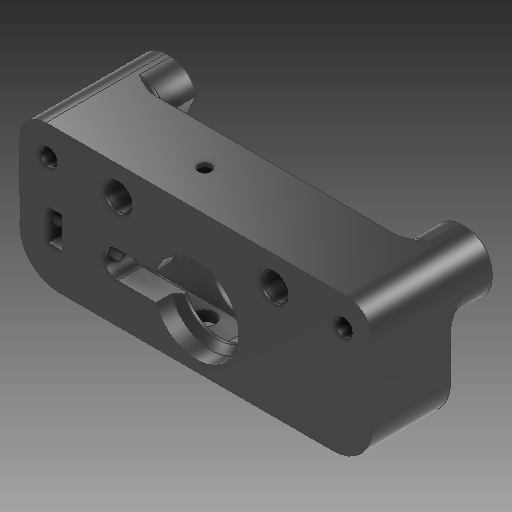
# Autodesk Inventor part: Extruder Clamp Block
Saved by Autodesk Inventor 2020.2 (Build 242310000, 310)
## iProperties
Created: 2020-03-19
Part Number: Extruder Clamp Block
Material: ABS Plastic
Document SubType Name: Modeling
Designer: rah75
Density: 1.06 g/cm^3
Appearance: Satin - Black
Author: rah75
Title: Upper Extruder Block
Autodesk Inventor part; units mm, degrees
ref_plane "YZ Plane" through (0, 0, 0) normal (1, 0, 0) x (0, 1, 0)
ref_plane "XZ Plane" through (0, 0, 0) normal (0, 1, 0) x (-1, 0, 0)
ref_plane "XY Plane" through (0, 0, 0) normal (0, 0, 1) x (1, 0, 0)
sketch "Sketch1" plane through (0, 0, 0) normal (0, 0, 1) x (1, 0, 0)
  line L0 (-28.9, 13) -> (28.9, 13)
  line L1 (33.9, 8) -> (33.9, -14)
  line L2 (33.9, -14) -> (-33.9, -14)
  line L3 (-33.9, -14) -> (-33.9, 8)
  arc A0 (33.9, 8) -> (28.9, 13) centre (28.9, 8) ccw
  arc A1 (-28.9, 13) -> (-33.9, 8) centre (-28.9, 8) ccw
  point P0 (0, 0)
  point P1 (-33.9, 13)
  point P2 (33.9, 13)
  point P3 (0, -14)
  point P4 (28.4, 7.5)
  point P5 (-28.4, 7.5)
  dimension "d2" = 27
  dimension "d72" = 67.8
  dimension "d73" = 5
  dimension "d74" = 57.8
  dimension "d75" = 14
  dimension "d76" = 5.5
  dimension "d77" = 5.5
  dimension "d78" = 5.5
  dimension "d79" = 5.5
  constraints: 8 end point, 4 point on circle, 4 point on line, 4 tangent, 2 centre point, 2 parallel, 1 equal radius, 1 horizontal, 1 midpoint, 1 perpendicular, 1 vertical alignment
  measures "d2" distance of L2.end point (-33.9, 13)
  measures "d72" distance of point (-33.9, 13) point (33.9, 13)
  measures "d73" radius of A0
  measures "d74" distance of A1.centre A0.centre
  measures "d75" distance from line of L2 point (0, 0)
  measures "d76" distance from line of L3 point (-28.4, 7.5)
  measures "d77" distance from line of L1 point (28.4, 7.5)
  measures "d78" distance from line of L0 point (28.4, 7.5)
  measures "d79" distance from line of L0 point (-28.4, 7.5)
extrude "Extrusion1" add sketch "Sketch1" along normal blind 15
fillet "Fillet1" radius 7.5 2 edges at (-33.9, -14, 7.5) (33.9, -14, 7.5)
sketch "Sketch10" plane through (0, 0, 0) normal (0, 0, -1) x (-1, 0, 0)
  arc A0 (-28.9, 13) -> (-33.9, 8) centre (-28.9, 8) ccw projected
  arc A1 (33.9, 8) -> (28.9, 13) centre (28.9, 8) ccw projected
  line L0 (-28.9, 13) -> (28.9, 13) projected
  line L1 (-33.9, -6.5) -> (-33.9, 8) projected
  line L2 (33.9, 8) -> (33.9, -6.5) projected
  point P0 (0, 0)
  point P1 (28.4, 7.5)
  point P2 (-28.4, 7.5)
  point P3 (-33.9, -13)
  point P4 (33.9, -13)
  dimension "d80" = 5.5
  dimension "d81" = 5.5
  dimension "d82" = 5.5
  dimension "d83" = 5.5
  measures "d80" distance from line of point (-28.4, 7.5) L0
  measures "d81" distance from line of L1 point (-28.4, 7.5)
  measures "d82" distance from line of point (28.4, 7.5) L0
  measures "d83" distance from line of L2 point (28.4, 7.5)
hole "Hole4" at (-28.4, 7.5, 0) at (28.4, 7.5, 0) direction (0, 0, 1) diameter 3.4 end through all clearance for "Socket Head Cap Screw" size "M3" standard "Ansi Metric M Profile"
sketch "Sketch2" plane through (-23.7815, 13, 0) normal (0, 1, 0) x (1, 0, 0)
  line L0 (52.6815, -15) -> (-5.1185, -15) projected
  point P0 (23.7815, 0)
  point P1 (17.6815, -7.25)
  dimension "d16" = 7.75
  dimension "d29" = 6.1
  measures "d16" distance from line of L0 point (17.682, -7.25)
  measures "d29" horizontal distance of point (17.682, -7.25) point (23.782, 0)
hole "Hole1" at (-6.1, 13, 7.25) direction (0, -1, 0) diameter 4 end through all
sketch "Sketch3" plane through (0, 0, 15) normal (0, 0, 1) x (1, 0, 0)
  circle A0 centre (0, -3.8) radius 7
  line L0 (33.9, -6.5) -> (33.9, 8) projected
  line L1 (28.9, 13) -> (-28.9, 13) projected
  point P0 (0, 0)
  point P1 (33.9, -1.1185)
  point P2 (21.2815, 11.5)
  point P3 (-21.2815, 11.5)
  point P4 (33.9, -13)
  dimension "d17" = 14
  dimension "d19" = 16.8
  constraints: 1 centre point, 1 vertical alignment, 1 other
  measures "d17" diameter of A0
extrude "Extrusion2" cut sketch "Sketch3" against normal blind 3.5
sketch "Sketch4" plane through (0, -3.8, 11.5) normal (0, 0, 1) x (1, 0, 0)
  circle A0 centre (0, 0) radius 7 projected
  point P0 (0, 3.8)
  point P1 (-4.2202, 6.2)
  point P2 (4.2202, 6.2)
  constraints: 1 coincident, 1 other
hole "Hole2" at (0, -3.8, 11.5) direction (0, 0, -1) diameter 11.5 end through all
sketch "Sketch5" plane through (0, 0, 0) normal (0, 0, -1) x (-1, 0, 0)
  circle A0 centre (0, -3.8) radius 5.75 projected
  line L0 (0, -3.8) -> (15.15, -3.8) construction
  line L1 (0, -6.425) -> (15.15, -6.425)
  line L2 (15.15, -1.175) -> (0, -1.175)
  arc A1 (0, -1.175) -> (0, -6.425) centre (0, -3.8) ccw
  arc A2 (15.15, -6.425) -> (15.15, -1.175) centre (15.15, -3.8) ccw
  point P0 (0, 0)
  point P1 (7.575, -3.8)
  dimension "d30" = 5.25
  dimension "d31" = 15.15
  constraints: 8 end point, 4 point on circle, 4 tangent, 2 centre point, 1 coincident, 1 horizontal, 1 midpoint, 1 parallel
  measures "d30" diameter of A2
  measures "d31" distance of L0.end A0.centre
extrude "Extrusion3" cut sketch "Sketch5" against normal through all contours A0 L1 A1 L2 | A0 L2 A2 L1 picked at (1.9167, -3.8)
sketch "Sketch6" plane through (0, 0, 0) normal (1, 0, 0) x (0, 1, 0)
  line L0 (-6.425, 15) -> (-1.175, 15) projected
  line L1 (-6.425, 0) -> (-6.425, 15) projected
  line L2 (-1.175, 0) -> (-6.425, 0) projected
  line L3 (-1.175, 0) -> (-1.175, 15) projected
  line L4 (4.45, 10.25) -> (-12.05, 10.25)
  line L5 (-12.05, 10.25) -> (-12.05, 4.25)
  line L6 (-12.05, 4.25) -> (4.45, 4.25)
  line L7 (4.45, 4.25) -> (4.45, 10.25)
  line L8 (4.45, 10.25) -> (-12.05, 4.25) construction
  line L9 (-12.05, 10.25) -> (4.45, 4.25) construction
  point P0 (0, 0)
  point P1 (-3.8, 7.25)
  point P2 (-3.8, 7.25)
  point P3 (-3.8, 0)
  dimension "d34" = 7.75
  dimension "d35" = 16.5
  dimension "d36" = 6
  constraints: 12 end point, 4 midpoint, 2 parallel, 1 horizontal, 1 perpendicular, 1 vertical alignment
  measures "d34" distance from line of L0 point (-3.8, 7.25)
  measures "d35" distance of L5.end L6.end
  measures "d36" distance of L6.end L4.start
extrude "Extrusion4" cut sketch "Sketch6" against normal blind 25 contours L4 L3 L6 L1 | L1 L6 L5 L4 | L4 L7 L6 L3
fillet "Fillet2" radius 8.25 2 edges at (-25, 4.45, 7.25) (-25, -12.05, 7.25)
sketch "Sketch7" plane through (0, 0, 0) normal (0, 0, -1) x (-1, 0, 0)
  arc A0 (5.1158, -1.175) -> (0, 1.95) centre (0, -3.8) ccw projected
  arc A1 (16.75, -12.05) -> (16.75, 4.45) centre (16.75, -3.8) ccw projected
  line L0 (0, 4.45) -> (16.75, 4.45) projected
  line L1 (0, 4.45) -> (0, 1.95) projected
  arc A2 (5.1158, -1.175) -> (0, 1.95) centre (0, -3.8) ccw projected
  line L2 (15.15, -1.175) -> (5.1158, -1.175) projected
  arc A3 (15.15, -6.425) -> (15.15, -1.175) centre (15.15, -3.8) ccw projected
  line L3 (5.1158, -6.425) -> (15.15, -6.425) projected
  arc A4 (0, -9.55) -> (5.1158, -6.425) centre (0, -3.8) ccw projected
  line L4 (0, -9.55) -> (0, -12.05) projected
  circle A5 centre (0, -3.8) radius 8.25
  line L5 (0, -12.05) -> (16.75, -12.05) projected
  point P0 (0, 0)
  constraints: 1 centre point, 1 coincident, 1 tangent
extrude "Extrusion5" cut sketch "Sketch7" against normal up to surface (10.25 mm away) contours L2 A5 L3 A4 L4 L1 A0 | A0 L1 A5 L2 | L4 A4 L3 A5
sketch "Sketch8" plane through (-33.9, -6.5, 0) normal (-1, 0, 0) x (0, 0, 1)
  line L0 (4.25, 0.075) -> (4.25, 5.325) projected
  line L1 (10.25, 5.325) -> (10.25, 0.075) projected
  line L2 (0, 0.075) -> (0, 5.325) projected
  line L3 (15, 5.325) -> (15, 0.075) projected
  line L4 (0, 2.7) -> (4.25, 2.7)
  line L5 (10.25, 2.7) -> (15, 2.7)
  point P0 (0, 6.5)
  point P1 (2.125, 2.7)
  point P2 (12.625, 2.7)
  point P3 (2.125, 2.7)
  point P4 (12.625, 2.7)
  constraints: 6 midpoint, 4 end point, 2 coincident, 2 horizontal
hole "Hole3" at (-33.9, -3.8, 2.125) at (-33.9, -3.8, 12.625) direction (1, 0, 0) diameter 3.2 end up to surface counterbore diameter 6.5 counterbore depth 0.1 clearance for "Socket Head Cap Screw" size "M3" standard "Ansi Metric M Profile"
sketch "Sketch9" plane through (0, 0, 0) normal (0, 0, -1) x (-1, 0, 0)
  line L0 (-28.9, 13) -> (28.9, 13) projected
  line L1 (-33.9, -6.5) -> (-33.9, 8) projected
  line L2 (26.4, -14) -> (-26.4, -14) projected
  arc A0 (7.8212, -1.175) -> (7.8212, -6.425) centre (0, -3.8) ccw projected
  line L3 (7.8212, -1.175) -> (15.15, -1.175) projected
  arc A1 (15.15, -6.425) -> (15.15, -1.175) centre (15.15, -3.8) ccw projected
  line L4 (15.15, -6.425) -> (7.8212, -6.425) projected
  line L5 (25.775, -0.8) -> (28.525, -0.8)
  line L6 (28.525, -0.8) -> (28.525, -6.8)
  line L7 (28.525, -6.8) -> (25.775, -6.8)
  line L8 (25.775, -6.8) -> (25.775, -0.8)
  line L9 (25.775, -0.8) -> (28.525, -6.8) construction
  line L10 (28.525, -0.8) -> (25.775, -6.8) construction
  line L11 (33.9, 8) -> (33.9, -1.341) projected
  arc A2 (33.9, 8) -> (28.9, 13) centre (28.9, 8) ccw projected
  arc A3 (-28.9, 13) -> (-33.9, 8) centre (-28.9, 8) ccw projected
  line L12 (33.8, -1.341) -> (33.9, -1.341) projected
  arc A4 (-33.9, -6.5) -> (-26.4, -14) centre (-26.4, -6.5) ccw projected
  arc A5 (26.4, -14) -> (33.9, -6.5) centre (26.4, -6.5) ccw projected
  line L13 (33.9, -6.259) -> (33.8, -6.259) projected
  line L14 (33.8, -6.259) -> (33.8, -1.341) projected
  line L15 (33.9, -6.259) -> (33.9, -6.5) projected
  point P0 (0, 0)
  point P1 (27.15, -3.8)
  point P2 (27.15, -3.8)
  point P3 (39.8, -3.8)
  point P4 (27.15, -3.8)
  dimension "d49" = 2.75
  dimension "d50" = 6
  dimension "d51" = 8
  constraints: 12 end point, 4 midpoint, 2 horizontal alignment, 2 parallel, 1 horizontal, 1 perpendicular
  measures "d49" distance of L5.start L5.end
  measures "d50" distance of L7.end L5.start
  measures "d51" distance edge to line of A1 L8
extrude "Extrusion6" cut sketch "Sketch9" against normal blind 21.1125 contours L5 L6 L7 L8
sketch "Sketch11" plane through (0, 0, 0) normal (0, 0, -1) x (-1, 0, 0)
  circle A0 centre (28.4, 7.5) radius 1.7 projected
  circle A1 centre (-28.4, 7.5) radius 1.7 projected
  line L0 (28.525, -0.8) -> (28.525, -6.8) projected
  line L1 (28.525, -6.8) -> (25.775, -6.8) projected
  line L2 (25.775, -6.8) -> (25.775, -0.8) projected
  line L3 (25.775, -0.8) -> (28.525, -0.8) projected
  line L4 (-28.9, 13) -> (28.9, 13) projected
  line L5 (-33.9, -6.5) -> (-33.9, 8) projected
  line L6 (26.4, -14) -> (-26.4, -14) projected
  arc A2 (7.8212, -1.175) -> (7.8212, -6.425) centre (0, -3.8) ccw projected
  line L7 (7.8212, -1.175) -> (15.15, -1.175) projected
  arc A3 (15.15, -6.425) -> (15.15, -1.175) centre (15.15, -3.8) ccw projected
  line L8 (15.15, -6.425) -> (7.8212, -6.425) projected
  circle A4 centre (-28.4, 7.5) radius 5.5
  circle A5 centre (28.4, 7.5) radius 1.7 projected
  circle A6 centre (28.4, 7.5) radius 5
  line L9 (33.9, 8) -> (33.9, -1.341) projected
  arc A7 (33.9, 8) -> (28.9, 13) centre (28.9, 8) ccw projected
  arc A8 (-28.9, 13) -> (-33.9, 8) centre (-28.9, 8) ccw projected
  line L10 (33.8, -1.341) -> (33.9, -1.341) projected
  arc A9 (-33.9, -6.5) -> (-26.4, -14) centre (-26.4, -6.5) ccw projected
  arc A10 (26.4, -14) -> (33.9, -6.5) centre (26.4, -6.5) ccw projected
  line L11 (33.9, -6.259) -> (33.8, -6.259) projected
  line L12 (33.8, -6.259) -> (33.8, -1.341) projected
  line L13 (22.9, 2) -> (33.9, 2)
  line L14 (33.9, 2) -> (33.9, 13)
  line L15 (33.9, 13) -> (22.9, 13)
  line L16 (22.9, 13) -> (22.9, 2)
  line L17 (22.9, 2) -> (33.9, 13) construction
  line L18 (33.9, 2) -> (22.9, 13) construction
  line L19 (33.9, 8) -> (33.9, -1.341) projected
  line L20 (-22.9, 2) -> (-33.9, 2)
  line L21 (-33.9, 2) -> (-33.9, 13)
  line L22 (-33.9, 13) -> (-22.9, 13)
  line L23 (-22.9, 13) -> (-22.9, 2)
  circle A11 centre (-28.4, 7.5) radius 1.7 projected
  line L24 (-22.9, 2) -> (-33.9, 13) construction
  line L25 (-33.9, 2) -> (-22.9, 13) construction
  line L26 (-33.9, -6.5) -> (-33.9, 8) projected
  line L27 (33.9, -6.259) -> (33.9, -6.5) projected
  point P0 (0, 0)
  point P1 (33.9, 8)
  point P2 (-22.9, 7.5)
  point P3 (-28.4, 13)
  point P4 (-28.4, 2)
  point P5 (-33.9, 7.5)
  point P6 (-33.9, 8)
  dimension "d61" = 11
  dimension "d62" = 10
  constraints: 24 end point, 4 collinear, 4 midpoint, 4 parallel, 2 centre point, 2 coincident, 2 horizontal, 2 perpendicular
  measures "d61" diameter of A4
  measures "d62" diameter of A6
extrude "Extrusion7" add sketch "Sketch11" along normal blind 8 contours L23 A4 L4 | L4 A7 L9 L13 L16 | A4 L5 A8 L4 | A4 | L23 L20 A4 | L15 L14 A7 | A8 L21 L22 | A4 L20 L5 | A6
fillet "Fillet4" radius 5 8 edges at (-33.9, 13, -4) (-22.9, 13, -4) (-33.9, 2, -4) (-22.9, 2, -4) (33.9, 13, -4) (33.9, 2, -4) (22.9, 2, -4) (22.9, 13, -4)
fillet "Fillet3" radius 2 10 edges at (22.9, 7.5, 0) (24.3645, 3.4645, 0) (28.4, 2, 0) (32.4355, 3.4645, 0) (24.3645, 11.5355, 0) (-24.3645, 11.5355, 0) (-24.3645, 3.4645, 0) (-28.4, 2, 0) (-32.4355, 3.4645, 0) (-22.9, 7.5, 0)
sketch "Sketch12" plane through (0, 0, 0) normal (0, 0, -1) x (-1, 0, 0)
  arc A0 (7.8212, -1.175) -> (7.8212, -6.425) centre (0, -3.8) ccw projected
  circle A1 centre (0, -3.8) radius 26.25
  dimension "d66" = 52.5
  constraints: 2 coincident, 1 centre point
  measures "d66" diameter of A1
extrude "Extrusion8" cut sketch "Sketch12" along normal blind 17.9375
sketch "Sketch13" plane through (0, 0, 15) normal (0, 0, 1) x (1, 0, 0)
  arc A0 (-5.1158, -6.425) -> (-5.1158, -1.175) centre (0, -3.8) ccw projected
  circle A1 centre (0, -3.8) radius 8.2
  point P0 (0, 0)
  dimension "d69" = 16.4
  constraints: 1 centre point, 1 coincident
  measures "d69" diameter of A1
extrude "Extrusion9" cut sketch "Sketch13" against normal blind 3
sketch "Sketch15" plane through (0, 0, 15) normal (0, 0, 1) x (1, 0, 0)
  circle A0 centre (-28.4, 7.5) radius 1.7 projected
  circle A1 centre (28.4, 7.5) radius 1.7 projected
  point P0 (0, 0)
  point P1 (-15, 7.5)
  point P2 (15, 7.5)
  dimension "d92" = 15
  dimension "d93" = 15
  constraints: 2 horizontal alignment
  measures "d92" horizontal distance of point (0, 0) point (-15, 7.5)
  measures "d93" horizontal distance of point (15, 7.5) point (0, 0)
hole "Hole7" at (-15, 7.5, 15) at (15, 7.5, 15) direction (0, 0, -1) diameter 5.5 depth 0.5
sketch "Sketch17" plane through (-15, 7.5, 14.5) normal (0, 0, 1) x (1, 0, 0)
  circle A0 centre (0, 0) radius 2.75 projected
  circle A1 centre (30, 0) radius 2.75 projected
  point P0 (15, -7.5)
  constraints: 2 coincident
hole "Hole8" at (-15, 7.5, 14.5) at (15, 7.5, 14.5) direction (0, 0, -1) diameter 5 depth 4.5 countersink diameter 5.4 countersink angle 8
sketch "Sketch18" plane through (0, 0, 15) normal (0, 0, 1) x (1, 0, 0)
  circle A0 centre (-15, 7.5) radius 2.75 projected
  circle A1 centre (15, 7.5) radius 2.75 projected
  point P0 (0, 0)
  constraints: 2 coincident
hole "Hole9" at (-15, 7.5, 15) at (15, 7.5, 15) direction (0, 0, -1) diameter 3.4 end through all clearance for "Socket Head Cap Screw" size "M3" standard "Ansi Metric M Profile"
sketch "Sketch19" plane through (0, 0, 11.5) normal (0, 0, 1) x (1, 0, 0)
  line L0 (-5.1158, -6.425) -> (-6.4892, -6.425) projected
  arc A0 (-6.4892, -6.425) -> (-6.4892, -1.175) centre (0, -3.8) ccw projected
  line L1 (-6.4892, -1.175) -> (-5.1158, -1.175) projected
  arc A1 (-5.1158, -6.425) -> (-5.1158, -1.175) centre (0, -3.8) ccw projected
  point P0 (0, 0)
extrude "Extrusion11" cut sketch "Sketch19" against normal through all
chamfer "Chamfer1" distance 0.75 angle 45 2 edges at (15, 9.2, 10) (-15, 9.2, 10)
sketch "Sketch20" plane through (-15.15, -3.8, 4.25) normal (0, 0, 1) x (1, 0, 0)
  arc A0 (15.15, 8.25) -> (7.3288, 2.625) centre (15.15, 0) ccw projected
  line L0 (15.15, 8.25) -> (-1.6, 8.25) projected
  arc A1 (-1.6, 8.25) -> (-1.6, -8.25) centre (-1.6, 0) ccw projected
  line L1 (15.15, -8.25) -> (-1.6, -8.25) projected
  arc A2 (7.3288, -2.625) -> (15.15, -8.25) centre (15.15, 0) ccw projected
  line L2 (0, -2.625) -> (7.3288, -2.625) projected
  arc A3 (0, 2.625) -> (0, -2.625) centre (0, 0) ccw projected
  line L3 (7.3288, 2.625) -> (0, 2.625) projected
  line L4 (15.15, 8.25) -> (15.15, -8.25)
  arc A4 (7.3288, -2.625) -> (15.15, -8.25) centre (15.15, 0) ccw projected
  point P0 (15.15, 3.8)
  constraints: 2 end point, 1 point on circle, 1 point on line
extrude "Extrusion12" [suppressed]
chamfer "Chamfer2" distance 1.2 angle 45 1 edges at (7, -3.8, 12)
sketch "Sketch21" plane through (-28.9, 13, 15) normal (0, 1, 0) x (1, 0, 0)
  circle A0 centre (22.8, 7.75) radius 2 projected
  circle A1 centre (22.8, 7.75) radius 1.25
  point P0 (28.9, 15)
  dimension "d139" = 0.75
  constraints: 1 centre point
  measures "d139" radial gap between concentric circles of A0 A1
extrude "Extrusion13" add sketch "Sketch21" against normal blind 0.75
equation "\"d78\" = d77"
equation "\"d79\" = d76"
body "Solid1"
